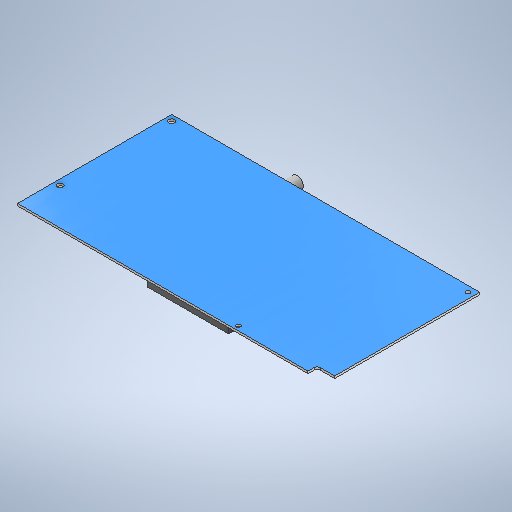
# Autodesk Inventor part: motherboard
Saved by Autodesk Inventor 2025.1 (Build 291241000, 241)
## iProperties
Created: 2024-09-23
Part Number: motherboard
Material: Generic
Document SubType Name: Modeling
Designer: PC
Density: 1 g/cm^3
Appearance: Default
Author: PC
Autodesk Inventor part; units mm, degrees
ref_plane "YZ Plane" through (0, 0, 0) normal (1, 0, 0) x (0, 1, 0)
ref_plane "XZ Plane" through (0, 0, 0) normal (0, 1, 0) x (-1, 0, 0)
ref_plane "XY Plane" through (0, 0, 0) normal (0, 0, 1) x (1, 0, 0)
sketch "Sketch1" plane through (0, 0, 0) normal (0, 1, 0) x (-1, 0, 0)
  line L0 (12, 105.1) -> (210, 105.1)
  line L1 (210, 105.1) -> (210, 0)
  line L2 (210, 0) -> (0, 0)
  circle A0 centre (4, 4) radius 1.5
  circle A1 centre (206, 4) radius 2
  circle A2 centre (206, 80.1) radius 2
  circle A3 centre (62.5, 102.1) radius 1.5
  line L3 (12, 105.1) -> (12, 100.9)
  line L4 (10, 98.9) -> (0, 98.9)
  arc A4 (10, 98.9) -> (12, 100.9) centre (10, 100.9) ccw
  line L5 (0, 98.9) -> (0, 0)
  point P0 (12, 98.9)
  dimension "d1" = 210
  dimension "d6" = 3
  dimension "d7" = 4
  dimension "d9" = 4
  dimension "d12" = 3
  dimension "d13" = 3
  dimension "d14" = 12
  dimension "d15" = 6.2
  dimension "d16" = 2
  dimension "d52" = 105.1
  dimension "d53" = 4
  dimension "d54" = 4
  dimension "d55" = 62.5
  dimension "d56" = 206
  dimension "d57" = 80.1
  dimension "d58" = 4
  constraints: 12 end point, 5 centre point, 2 horizontal, 2 point on circle, 2 point on line, 2 tangent, 2 vertical, 1 coincident, 1 parallel, 1 perpendicular, 1 vertical alignment
  measures "d1" distance of L1.end L2.end
  measures "d6" diameter of A0
  measures "d7" diameter of A1
  measures "d9" diameter of A2
  measures "d12" distance from line of L0 A3.centre
  measures "d13" diameter of A3
  measures "d14" distance of point (12, 98.9) L4.end
  measures "d15" distance of L0.start point (12, 98.9)
  measures "d16" radius of A4
  measures "d52" distance between parallel lines of L0 L2
  measures "d53" distance from line of L2 A0.centre
  measures "d54" distance from line of L5 A0.centre
  measures "d55" distance from line of L5 A3.centre
  measures "d56" distance from line of L5 A1.centre
  measures "d57" distance from line of L2 A2.centre
  measures "d58" distance from line of L2 A1.centre
extrude "Extrusion1" add sketch "Sketch1" along normal blind 1.5
sketch "Sketch2" plane through (0, 0, 0) normal (0, -1, 0) x (1, 0, 0)
  line L0 (-126.75, 100.1) -> (-71.15, 100.1)
  line L1 (-71.15, 100.1) -> (-71.15, 95.6)
  line L2 (-71.15, 95.6) -> (-126.75, 95.6)
  line L3 (-126.75, 95.6) -> (-126.75, 100.1)
  line L4 (-210, 0) -> (-210, 105.1) projected
  line L5 (0, 98.9) -> (0, 0) projected
  line L6 (-72.7, 96.85) -> (-125.2, 96.85)
  line L7 (-125.2, 96.85) -> (-125.2, 98.85)
  line L8 (-125.2, 98.85) -> (-72.7, 98.85)
  line L9 (-72.7, 98.85) -> (-72.7, 96.85)
  line L10 (-210, 105.1) -> (-12, 105.1) projected
  point P0 (-126.75, 97.85)
  point P1 (-72.7, 97.85)
  point P2 (-71.15, 97.85)
  point P3 (-98.95, 98.85)
  point P4 (-98.95, 100.1)
  point P5 (-111, 105.1)
  dimension "d17" = 4.5
  dimension "d18" = 55.6
  dimension "d33" = 52.5
  dimension "d34" = 2
  dimension "d35" = 71.15
  dimension "d36" = 5
  constraints: 16 end point, 6 midpoint, 4 parallel, 2 horizontal, 2 perpendicular, 1 horizontal alignment, 1 vertical alignment
  measures "d17" distance between parallel lines of L2 L0
  measures "d18" distance of L1.end L2.end
  measures "d33" distance of L6.start L6.end
  measures "d34" distance between parallel lines of L8 L6
  measures "d35" distance from line of L5 L0.end
  measures "d36" distance from line of point (-111, 105.1) L0
sketch "Sketch3" plane through (0, 0, 0) normal (0, -1, 0) x (1, 0, 0)
  line L0 (0, 0) -> (-210, 0) projected
  line L1 (-55.6, 0) -> (-86.6, 0)
  line L2 (-86.6, 0) -> (-86.6, 16)
  line L3 (-86.6, 16) -> (-55.6, 16)
  line L4 (-55.6, 16) -> (-55.6, 0)
  line L5 (0, 98.9) -> (0, 0) projected
  point P0 (-55.6, 8)
  point P1 (-86.6, 0)
  dimension "d23" = 55.6
  dimension "d24" = 31
  dimension "d25" = 16
  constraints: 8 end point, 2 parallel, 1 horizontal, 1 midpoint, 1 perpendicular, 1 point on line
  measures "d23" distance from line of L5 point (-55.6, 8)
  measures "d24" distance of L2.end L3.end
  measures "d25" distance of L1.end L2.end
extrude "Extrusion3" add sketch "Sketch3" along normal blind 12.5
sketch "Sketch4" plane through (0, 0, 0) normal (0, -1, 0) x (1, 0, 0)
  line L0 (-106.2, 0) -> (-120.2, 0)
  line L1 (-120.2, 0) -> (-120.2, 12.75)
  line L2 (-120.2, 12.75) -> (-106.2, 12.75)
  line L3 (-106.2, 12.75) -> (-106.2, 0)
  line L4 (-86.6, 16) -> (-86.6, 0) projected
  line L5 (0, 0) -> (-55.6, 0) projected
  line L6 (-86.6, 0) -> (-210, 0) projected
  dimension "d28" = 12.75
  dimension "d29" = 14
  dimension "d32" = 19.6
  constraints: 8 end point, 2 parallel, 1 collinear, 1 horizontal, 1 perpendicular
  measures "d28" distance of L0.end L1.end
  measures "d29" distance of L1.end L2.end
  measures "d32" distance between parallel lines of L4 L3
extrude "Extrusion4" add sketch "Sketch4" along normal blind 13.15
extrude "Extrusion5" add sketch "Sketch2" along normal blind 8.6
sketch "Sketch5" plane through (0, 0, 0) normal (0, -1, 0) x (1, 0, 0)
  line L0 (0, 0) -> (-210, 0) projected
  line L1 (-185, 0) -> (-173.5, 0)
  line L2 (-173.5, 0) -> (-173.5, 17)
  line L3 (-173.5, 17) -> (-185, 17)
  line L4 (-185, 17) -> (-185, 0)
  line L5 (-210, 0) -> (-210, 105.1) projected
  point P0 (-173.5, 0)
  dimension "d39" = 17
  dimension "d40" = 11.5
  dimension "d43" = 25
  constraints: 8 end point, 2 parallel, 1 horizontal, 1 perpendicular, 1 point on line
  measures "d39" distance of L3.end L1.start
  measures "d40" distance of L2.end L3.end
  measures "d43" distance between parallel lines of L5 L4
extrude "Extrusion6" add sketch "Sketch5" along normal blind 11
sketch "Sketch6" plane through (0, 0, 0) normal (0, -1, 0) x (1, 0, 0)
  line L0 (0, 0) -> (-210, 0) projected
  line L1 (-139.4357, 0) -> (-129.4357, 0)
  line L2 (-129.4357, 0) -> (-129.4357, 10)
  line L3 (-129.4357, 10) -> (-139.4357, 10)
  line L4 (-139.4357, 10) -> (-139.4357, 0)
  point P0 (-129.4357, 0)
  dimension "d44" = 10
  dimension "d45" = 10
  constraints: 8 end point, 2 parallel, 1 horizontal, 1 perpendicular, 1 point on line
  measures "d44" distance of L2.end L3.end
  measures "d45" distance of L3.end L1.start
extrude "Extrusion7" add sketch "Sketch6" along normal blind 12
sketch "Sketch7" plane through (0, 1.5, 0) normal (0, 0, -1) x (-1, 0, 0)
  circle A0 centre (134.4357, -7.5) radius 4.15
  line L0 (139.4357, -1.5) -> (139.4357, -13.5) projected
  line L1 (139.4357, -13.5) -> (129.4357, -13.5) projected
  point P0 (0, -1.5)
  point P1 (139.4357, -7.5)
  point P2 (134.4357, -13.5)
  dimension "d48" = 8.3
  constraints: 2 midpoint, 1 centre point, 1 horizontal alignment, 1 vertical alignment
  measures "d48" diameter of A0
extrude "Extrusion8" add sketch "Sketch7" along normal blind 10
body "Solid1"
